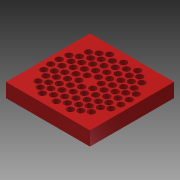
# Autodesk Inventor part: FanTemplate60mm
Saved by Autodesk Inventor 2015 SP1 (Build 190203100, 203)
## iProperties
Created: 2015-04-15
Part Number: FanTemplate60mm
Material: Generic
Document SubType Name: Modeling
Designer: Jack
Density: 1 g/cm^3
Appearance: Light Red
Author: Jack
Autodesk Inventor part; units mm, degrees
ref_plane "YZ Plane" through (0, 0, 0) normal (1, 0, 0) x (0, 1, 0)
ref_plane "XZ Plane" through (0, 0, 0) normal (0, 1, 0) x (-1, 0, 0)
ref_plane "XY Plane" through (0, 0, 0) normal (0, 0, 1) x (1, 0, 0)
sketch "Sketch1" plane through (0, 0, 0) normal (0, 0, 1) x (1, 0, 0)
  line L0 (-30, -30) -> (30, -30)
  line L1 (30, -30) -> (30, 30)
  line L2 (30, 30) -> (-30, 30)
  line L3 (-30, 30) -> (-30, -30)
  line L4 (-30, -30) -> (30, 30) construction
  line L5 (30, -30) -> (-30, 30) construction
  point P0 (0, 0)
  dimension "d0" = 60
  dimension "d1" = 60
  constraints: 12 end point, 2 midpoint, 2 parallel, 1 horizontal, 1 perpendicular
  measures "d0" distance of L2.end L1.end
  measures "d1" distance of L1.end L0.end
extrude "Extrusion1" add sketch "Sketch1" along normal blind 10
sketch "Sketch2" plane through (0, 0, 10) normal (0, 0, 1) x (1, 0, 0)
  circle A0 centre (0, 0) radius 29
  line L0 (-20, 21) -> (20, 21) construction
  line L1 (-22.7376, 18) -> (22.7376, 18) construction
  line L2 (-24.8193, 15) -> (24.8193, 15) construction
  line L3 (-26.4008, 12) -> (-26.4008, 12) construction
  line L4 (-26.4008, 12) -> (26.4008, 12) construction
  line L5 (-27.5681, 9) -> (27.5681, 9) construction
  line L6 (-10.583, 27) -> (10.583, 27) construction
  line L7 (-16.2788, 24) -> (16.2788, 24) construction
  line L8 (-28.3725, 6) -> (28.3725, 6) construction
  line L9 (-28.8444, 3) -> (28.8444, 3) construction
  line L10 (-29, 0) -> (29, 0) construction
  circle A1 centre (0, 24) radius 2.38
  circle A2 centre (-10, 24) radius 2.38
  circle A3 centre (10, 24) radius 2.38
  circle A4 centre (5, 21) radius 2.38
  circle A5 centre (14.5, 21) radius 2.38
  circle A6 centre (-5, 21) radius 2.38
  circle A7 centre (-14.5, 21) radius 2.38
  circle A8 centre (-10, 18) radius 2.38
  circle A9 centre (-19, 18) radius 2.38
  circle A10 centre (0, 18) radius 2.38
  circle A11 centre (10, 18) radius 2.38
  circle A12 centre (19, 18) radius 2.38
  circle A13 centre (-14.5, 15) radius 2.38
  circle A14 centre (-5, 15) radius 2.38
  circle A15 centre (5, 15) radius 2.38
  circle A16 centre (14.5, 15) radius 2.38
  circle A17 centre (-19.5, 12) radius 2.38
  circle A18 centre (-10, 12) radius 2.38
  circle A19 centre (0, 12) radius 2.38
  circle A20 centre (10, 12) radius 2.38
  circle A21 centre (19.5, 12) radius 2.38
  circle A22 centre (-24, 9) radius 2.38
  circle A23 centre (-15, 9) radius 2.38
  circle A24 centre (-5, 9) radius 2.38
  circle A25 centre (5, 9) radius 2.38
  circle A26 centre (15, 9) radius 2.38
  circle A27 centre (24, 9) radius 2.38
  circle A28 centre (-19.5, 6) radius 2.38
  circle A29 centre (-10, 6) radius 2.38
  circle A30 centre (0, 6) radius 2.38
  circle A31 centre (10, 6) radius 2.38
  circle A32 centre (19.5, 6) radius 2.38
  circle A33 centre (-25, 3) radius 2.38
  circle A34 centre (-15, 3) radius 2.38
  circle A35 centre (-5, 3) radius 2.38
  circle A36 centre (5, 3) radius 2.38
  circle A37 centre (15, 3) radius 2.38
  circle A38 centre (25, 3) radius 2.38
  circle A39 centre (-20, 0) radius 2.38
  circle A40 centre (-10, 0) radius 2.38
  circle A41 centre (10, 0) radius 2.38
  circle A42 centre (20, 0) radius 2.38
  dimension "d4" = 58
  dimension "d5" = 3
  dimension "d6" = 3
  dimension "d7" = 3
  dimension "d8" = 3
  dimension "d9" = 3
  dimension "d10" = 3
  dimension "d11" = 3
  dimension "d12" = 3
  dimension "d13" = 3
  dimension "d14" = 4.76
  dimension "d15" = 10
  dimension "d16" = 10
  dimension "d17" = 14.5
  dimension "d18" = 5
  dimension "d19" = 5
  dimension "d20" = 14.5
  dimension "d21" = 10
  dimension "d22" = 19
  dimension "d23" = 19
  dimension "d24" = 10
  dimension "d25" = 5
  dimension "d26" = 5
  dimension "d27" = 14.5
  dimension "d28" = 14.5
  dimension "d29" = 10
  dimension "d30" = 10
  dimension "d31" = 19.5
  dimension "d32" = 19.5
  dimension "d33" = 24
  dimension "d34" = 24
  dimension "d35" = 15
  dimension "d36" = 15
  dimension "d37" = 5
  dimension "d38" = 5
  dimension "d39" = 5
  dimension "d40" = 5
  dimension "d41" = 15
  dimension "d42" = 25
  dimension "d43" = 25
  dimension "d44" = 15
  dimension "d45" = 20
  dimension "d46" = 10
  dimension "d47" = 10
  dimension "d48" = 20
  constraints: 42 centre point, 41 equal radius, 39 point on line, 22 end point, 6 parallel, 5 vertical alignment, 4 horizontal, 4 midpoint, 1 coincident, 1 horizontal alignment, 22 other
  measures "d5" distance between parallel lines of L4 L5
  measures "d6" distance between parallel lines of L4 L2
  measures "d7" distance between parallel lines of L1 L2
  measures "d8" distance between parallel lines of L0 L1
  measures "d9" distance between parallel lines of L8 L9
  measures "d10" distance between parallel lines of L5 L8
  measures "d11" distance between parallel lines of L7 L0
  measures "d12" distance between parallel lines of L6 L7
  measures "d13" distance between parallel lines of L9 L10
  measures "d14" diameter of A1
  measures "d15" distance of A1.centre A3.centre
  measures "d16" distance of A1.centre A2.centre
  measures "d17" horizontal distance of A1.centre A7.centre
  measures "d18" horizontal distance of A6.centre A1.centre
  measures "d19" horizontal distance of A1.centre A4.centre
  measures "d20" horizontal distance of A5.centre A1.centre
  measures "d21" distance of A10.centre A8.centre
  measures "d22" distance of A10.centre A9.centre
  measures "d23" distance of A10.centre A12.centre
  measures "d24" distance of A10.centre A11.centre
  measures "d25" horizontal distance of A10.centre A14.centre
  measures "d26" horizontal distance of A10.centre A15.centre
  measures "d27" horizontal distance of A10.centre A13.centre
  measures "d28" horizontal distance of A16.centre A10.centre
  measures "d29" distance of A19.centre A20.centre
  measures "d30" distance of A19.centre A18.centre
  measures "d31" distance of A19.centre A17.centre
  measures "d32" distance of A19.centre A21.centre
  measures "d33" horizontal distance of A19.centre A22.centre
  measures "d34" horizontal distance of A27.centre A19.centre
  measures "d35" horizontal distance of A19.centre A26.centre
  measures "d36" horizontal distance of A19.centre A23.centre
  measures "d37" horizontal distance of A19.centre A24.centre
  measures "d38" horizontal distance of A19.centre A25.centre
  measures "d39" horizontal distance of A30.centre A35.centre
  measures "d40" horizontal distance of A36.centre A30.centre
  measures "d41" horizontal distance of A37.centre A30.centre
  measures "d42" horizontal distance of A30.centre A38.centre
  measures "d43" horizontal distance of A30.centre A33.centre
  measures "d44" horizontal distance of A30.centre A34.centre
  measures "d45" distance of point (0, 0) A39.centre
  measures "d46" distance of point (0, 0) A40.centre
  measures "d47" distance of point (0, 0) A41.centre
  measures "d48" distance of A42.centre point (0, 0)
extrude "Extrusion2" cut sketch "Sketch2" against normal up to next contours A1 | A2 | A3 | A4 | A5 | A6 | A7 | A8 | A9 | A10 | A11 | A12 | A13 | A14 | A15 | A16 | A17 | A18 | A19 | A20 | A21 | A22 | A23 | A24 | A25 | A26 | A27 | A28 | A29 | A30 | A31 | A32 | A33 | A34 | A35 | A36 | A37 | A38 | A39 | A40 | A41 | A42
ref_plane "Work Plane1" through (-30, 0, 0) normal (0, 1, 0) x (1, 0, 0)
mirror "Mirror1" about plane through (-30, 0, 0) normal (0, 1, 0) of "Extrusion2"
body "Solid1"
